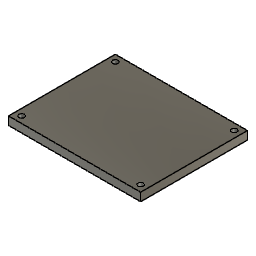
PCB Mount v1 (Autodesk Fusion 360 design; units mm, degrees)
Autodesk Fusion 360 part; units mm, degrees
sketch "Sketch1" plane through (0, 0, 0) normal (0, 0, 1) x (1, 0, 0)
  circle A0 centre (36.1, -17.1) radius 1.65
  line L0 (-40.064, 43.7) -> (-40.064, -21.1)
  circle A1 centre (36.1, -17.1) radius 1.65
  circle A2 centre (-36.064, 39.7) radius 1.65
  line L1 (-40.064, -21.1) -> (40.1, -21.1)
  circle A3 centre (36.1, 39.7) radius 1.65
  circle A4 centre (-36.064, -17.1) radius 1.65
  line L2 (40.1, -21.1) -> (40.1, 43.7)
  circle A5 centre (-36.064, 39.7) radius 1.65
  line L3 (-40.064, -21.1) -> (-40.064, 43.7)
  circle A6 centre (36.1, 39.7) radius 1.65
  circle A7 centre (-36.064, -17.1) radius 1.65
  line L4 (40.1, 43.7) -> (40.1, -21.1)
  line L5 (40.1, 43.7) -> (-40.064, 43.7)
  constraint coincident L0.end L1.start
  constraint coincident L0.start L3.end
  constraint coincident L2.end L4.start
  constraint coincident L1.end L2.start
  constraint concentric A0 A1
  constraint concentric A4 A7
  constraint concentric A2 A5
  constraint concentric A3 A6
extrude "Extrude1" add sketch "Sketch1" along normal blind 5
